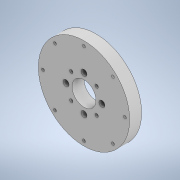
# Autodesk Inventor part: Roue
Saved by Autodesk Inventor 2020.1 (Build 241239000, 239)
## iProperties
Created: 2019-11-14
Part Number: Roue
Material: Generic
Document SubType Name: Modeling
Designer: Admin
Density: 1 g/cm^3
Appearance: Default
Author: Admin
Autodesk Inventor part; units mm, degrees
ref_plane "YZ Plane" through (0, 0, 0) normal (1, 0, 0) x (0, 1, 0)
ref_plane "XZ Plane" through (0, 0, 0) normal (0, 1, 0) x (-1, 0, 0)
ref_plane "XY Plane" through (0, 0, 0) normal (0, 0, 1) x (1, 0, 0)
sketch "Sketch1" plane through (0, 0, 0) normal (0, 0, 1) x (1, 0, 0)
  circle A0 centre (0, 0) radius 48.514
  circle A1 centre (0, 0) radius 12.7
  circle A2 centre (0, 0) radius 19.05
  circle A3 centre (0, 19.05) radius 3.175
  circle A4 centre (-19.05, 0) radius 3.175
  circle A5 centre (0, -19.05) radius 3.175
  circle A6 centre (19.05, 0) radius 3.175
  circle A7 centre (-13.4704, 13.4704) radius 1.778
  circle A8 centre (13.4704, 13.4704) radius 1.778
  circle A9 centre (13.4704, -13.4704) radius 1.778
  circle A10 centre (-13.4704, -13.4704) radius 1.778
  line L0 (0, 0) -> (13.4704, 13.4704)
  line L1 (0, 0) -> (19.05, 0)
  line L2 (13.4704, -13.4704) -> (0, 0)
  line L3 (0, 0) -> (0, -19.05)
  line L4 (-13.4704, -13.4704) -> (0, 0)
  circle A11 centre (0, 0) radius 43.5229
  circle A12 centre (-43.5229, 0) radius 1.524
  circle A13 centre (-30.7753, 30.7753) radius 1.524
  circle A14 centre (0, 43.5229) radius 1.524
  circle A15 centre (30.7753, 30.7753) radius 1.524
  circle A16 centre (43.5229, 0) radius 1.524
  circle A17 centre (30.7753, -30.7753) radius 1.524
  circle A18 centre (0, -43.5229) radius 1.524
  circle A19 centre (-30.7753, -30.7753) radius 1.524
  line L5 (-43.5229, 0) -> (0, 0)
  dimension "d3" = 38.1
  dimension "d17" = 87.0458
  dimension "d1" = 97.028
  dimension "d2" = 25.4
  dimension "d4" = 6.35
  dimension "d5" = 6.35
  dimension "d6" = 6.35
  dimension "d7" = 6.35
  dimension "d8" = 3.556
  dimension "d9" = 3.556
  dimension "d10" = 3.556
  dimension "d11" = 3.556
  dimension "d14" = 45
  dimension "d15" = 45
  dimension "d16" = 45
  dimension "d18" = 3.048
  dimension "d19" = 3.048
  dimension "d20" = 3.048
  dimension "d21" = 3.048
  dimension "d22" = 3.048
  dimension "d23" = 3.048
  dimension "d24" = 3.048
  dimension "d25" = 3.048
  constraints: 18 centre point, 12 end point, 3 coincident, 2 horizontal, 2 perpendicular, 2 point on line, 20 other
  measures "d1" diameter of A0
  measures "d2" diameter of A1
  measures "d4" diameter of A3
  measures "d5" diameter of A6
  measures "d6" diameter of A4
  measures "d7" diameter of A5
  measures "d8" diameter of A7
  measures "d9" diameter of A8
  measures "d10" diameter of A9
  measures "d11" diameter of A10
  measures "d14" angle of L1 L0
  measures "d15" angle of L2 L1
  measures "d16" angle of L4 L3
  measures "d18" diameter of A12
  measures "d19" diameter of A13
  measures "d20" diameter of A14
  measures "d21" diameter of A15
  measures "d22" diameter of A16
  measures "d23" diameter of A17
  measures "d24" diameter of A18
  measures "d25" diameter of A19
extrude "Extrusion1" add sketch "Sketch1" along normal blind 12.7 contours A0 | L1 A6 A2 A9 L2 A1 | A1 L0 A8 A2 A6 L1 | A1 L5 A4 A2 A7 A3 A8 L0 | L2 A9 A2 A5 L3 A1 | A1 L4 A10 A2 A4 L5 | L3 A5 A2 A10 L4 A1 | A12 A11 A13 A14 A15 A16 A17 A18 A19
body "Solid1"
